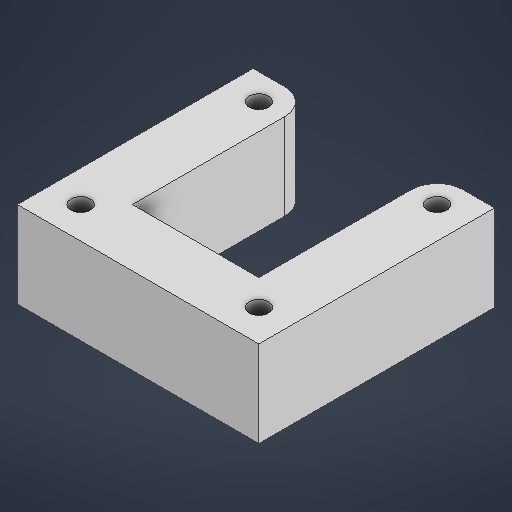
# Autodesk Inventor part: MOTOR standoff
Saved by Autodesk Inventor 2025.1 (Build 291241000, 241)
## iProperties
Created: 2025-02-02
Part Number: MOTOR standoff
Material: Generic
Document SubType Name: Modeling
Designer: jerem
Density: 1 g/cm^3
Appearance: Default
Author: jerem
Autodesk Inventor part; units mm, degrees
ref_plane "YZ Plane" through (0, 0, 0) normal (1, 0, 0) x (0, 1, 0)
ref_plane "XZ Plane" through (0, 0, 0) normal (0, 1, 0) x (-1, 0, 0)
ref_plane "XY Plane" through (0, 0, 0) normal (0, 0, 1) x (1, 0, 0)
sketch "Sketch2" plane through (0, 0, 0) normal (0, 1, 0) x (-1, 0, 0)
  line L0 (21, -21) -> (-21, -21)
  line L1 (-21, -21) -> (-21, 21)
  line L2 (-21, 21) -> (21, 21)
  line L3 (21, 21) -> (21, -21)
  line L4 (21, -21) -> (-21, 21) construction
  line L5 (-21, -21) -> (21, 21) construction
  circle A0 centre (-15.5, 15.5) radius 1.7
  circle A1 centre (15.5, 15.5) radius 1.7
  circle A2 centre (15.5, -15.5) radius 1.7
  circle A3 centre (-15.5, -15.5) radius 1.7
  line L6 (-15.5, 15.5) -> (-15.5, -15.5) construction
  line L7 (-15.5, 15.5) -> (15.5, 15.5) construction
  line L8 (15.5, 15.5) -> (15.5, -15.5) construction
  circle A4 centre (-15.5, 15.5) radius 4.5
  circle A5 centre (15.5, 15.5) radius 4.5
  circle A6 centre (15.5, -15.5) radius 4.5
  circle A7 centre (-15.5, -15.5) radius 4.5
  circle A8 centre (0, 0) radius 10
  line L9 (11, -15.5) -> (11, 11)
  line L10 (11, 11) -> (-11, 11)
  line L11 (-11, 11) -> (-11, -15.5)
  line L12 (-15.5, -20) -> (-21, -20)
  line L13 (15.5, -20) -> (21, -20)
  dimension "d4" = 42
  dimension "d5" = 42
  dimension "d6" = 31
  dimension "d7" = 3.4
  dimension "d9" = 20
  dimension "d12" = 9
  constraints: 28 end point, 10 point on line, 9 centre point, 6 equal radius, 4 perpendicular, 4 point on circle, 3 parallel, 3 tangent, 2 coincident, 2 midpoint, 2 vertical, 1 horizontal
  measures "d4" distance of L2.start L2.end
  measures "d5" distance of L0.end L2.start
  measures "d6" distance of L7.start L8.start
  measures "d7" diameter of A0
  measures "d9" diameter of A8
  measures "d12" diameter of A5
extrude "Extrusion2" add sketch "Sketch2" along normal blind 15 contours L13 A6 L9 L10 L11 A7 L12 L1 L2 L3 | A6 | A7 | A4 | A5
body "Solid2"
